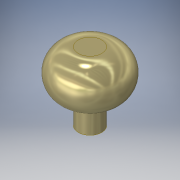
# Autodesk Inventor part: Part1
Saved by Autodesk Inventor 2016 (Build 200138000, 138)
## iProperties
Created: 2017-02-28
Part Number: Part1
Material: Generic
Document SubType Name: Modeling
Designer: caleb
Density: 1 g/cm^3
Appearance: Gold - Metal
Author: caleb
Autodesk Inventor part; units mm, degrees
ref_plane "YZ Plane" through (0, 0, 0) normal (1, 0, 0) x (0, 1, 0)
ref_plane "XZ Plane" through (0, 0, 0) normal (0, 1, 0) x (-1, 0, 0)
ref_plane "XY Plane" through (0, 0, 0) normal (0, 0, 1) x (1, 0, 0)
sketch "Sketch1" plane through (0, 0, 0) normal (0, 0, 1) x (1, 0, 0)
  line L0 (-6.35, 3.5318) -> (0, 0)
  line L1 (0, 0) -> (0, 7.4744)
  line L2 (0, 7.4744) -> (-6.35, 7.6046)
  line L3 (-6.35, 7.6046) -> (-6.35, 16.5736)
  arc A0 (-6.35, 40.5512) -> (-6.35, 16.5736) centre (-6.5757, 28.5624) ccw
  line L4 (-6.35, 40.5512) -> (0, 40.5512)
  line L5 (0, 40.5512) -> (0, 7.4744)
  line L6 (-6.35, 7.6046) -> (-6.35, 3.5318)
  constraints: 14 end point, 3 vertical, 2 point on circle, 1 centre point, 1 horizontal, 1 perpendicular
revolve "Revolution1" add sketch "Sketch1" angle 360 about axis through (0, 40.5512, 0) along (0, -1, 0)
body "Solid1"
